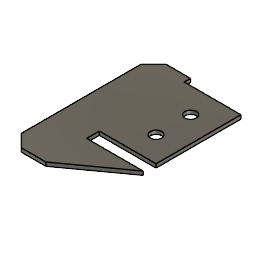
GPL H250 to H175G11 (Autodesk Fusion 360 design; units mm, degrees)
Autodesk Fusion 360 part; units mm, degrees
sketch "スケッチ1" plane through (0, 0, 0) normal (0, 0, 1) x (1, 0, 0)
  line L0 (-15.5, 115) -> (-74.5, 115)
  line L1 (-74.5, 115) -> (-74.5, -115)
  line L2 (-74.5, -115) -> (-15.5, -115)
  line L3 (74.5, -30) -> (74.5, 105)
  line L4 (68.0217, 105) -> (-74.5, -115) construction
  line L5 (-74.5, 115) -> (45.8131, -70.7183) construction
  line L6 (-15.5, 115) -> (-15.5, 105)
  line L7 (-15.5, 105) -> (74.5, 105)
  line L8 (-74.5, -115) -> (-15.5, -115) construction
  line L9 (74.5, -50) -> (-15.5, -115)
  line L10 (74.5, -50) -> (-15.5, -50)
  line L11 (-15.5, -50) -> (-15.5, -30)
  line L12 (-15.5, -30) -> (74.5, -30)
  dimension "d2" = 230
  dimension "d5" = 59
  dimension "d7" = 90
  dimension "d8" = 20
  constraint horizontal L0
  constraint perpendicular L0 L1
  constraint parallel L0 L2
  constraint parallel L1 L3
  constraint coincident L4 origin
  constraint coincident L5 origin
  constraint vertical L6
  constraint horizontal L7
  constraint coincident L7 L4.start
  constraint perpendicular L1 L8
  constraint coincident L9 L5.end
  constraint horizontal L10
  constraint vertical L11
  constraint horizontal L12
  measures "d2" distance of L0.end L1.end
  measures "d5" distance of L1.end L2.end
  measures "d7" distance of L9.start L10.end
  measures "d8" distance of L9.start L3.start
extrude "押し出し1" add sketch "スケッチ1" along normal blind 6
chamfer "面取り1" distance 20 angle 45 2 edges at (-74.5, -115, 3) (-74.5, 115, 3)
sketch "スケッチ2" plane through (0, 0, 6) normal (0, 0, 1) x (-1, 0, 0)
  line L0 (54.5, -115) -> (74.5, -95)
  line L1 (74.5, -95) -> (74.5, 95)
  line L2 (74.5, 95) -> (54.5, 115)
  line L3 (54.5, 115) -> (15.5, 115)
  line L4 (15.5, 115) -> (-74.5, 50)
  line L5 (-74.5, 50) -> (15.5, 50)
  line L6 (15.5, 50) -> (15.5, 30)
  line L7 (15.5, 30) -> (-74.5, 30)
  line L8 (-74.5, 30) -> (-74.5, -105)
  line L9 (-74.5, -105) -> (15.5, -105)
  line L10 (15.5, -105) -> (15.5, -115)
  line L11 (15.5, -115) -> (54.5, -115)
  line L12 (-74.5, -105) -> (-34.5, -105) construction
  line L13 (-34.5, -105) -> (-34.5, -65) construction
  line L14 (-34.5, -65) -> (-74.5, -65) construction
  line L15 (-74.5, -65) -> (-74.5, -105) construction
  line L16 (-34.5, -65) -> (-34.5, -10) construction
  point P0 (-34.5, -65)
  point P1 (-34.5, -10)
  dimension "d12" = 40
  dimension "d13" = 40
  dimension "d14" = 55
  constraint horizontal L12
  constraint vertical L13
  constraint horizontal L14
  constraint vertical L15
  constraint coincident L8.end L9.start
  constraint perpendicular L14 L16
  constraint coincident P0 L13.end
  constraint coincident P1 L16.end
  measures "d12" distance of L8.end L12.end
  measures "d13" distance of L8.end L14.end
  measures "d14" distance of P0 P1
hole "穴1" at (34.5, 65, 6) at (34.5, 10, 6) direction (0, 0, -1) diameter 18 end through all
equation "d5 = 20 mm + 39 mm"
